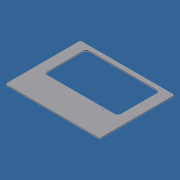
# Autodesk Inventor part: P1699_002_FaceAvant
Saved by Autodesk Inventor 2015 SP2 (Build 190223200, 223)
## iProperties
Created: 2017-01-26
Part Number: P1699_002_FaceAvant
Project: Nom Projet
Material: .
Description: Nom pièce
Document SubType Name: Modeling
Designer: Jean-Marc.VULLIAMY
Authority: brut Ø
Density: 1 g/cm^3
Appearance: Par défaut(1)
Mass: 77.5499 g
Surface Area: 565.1 cm^2
Volume: 77.5499 cm^3
Material number: ---
Author: Jean-Marc.VULLIAMY
Autodesk Inventor part; units mm, degrees
ref_plane "Plan YZ" through (0, 0, 0) normal (1, 0, 0) x (0, 1, 0)
ref_plane "Plan XZ" through (0, 0, 0) normal (0, 1, 0) x (-1, 0, 0)
ref_plane "Plan XY" through (0, 0, 0) normal (0, 0, 1) x (1, 0, 0)
sketch "Esquisse1" plane through (0, 0, 0) normal (0, 0, 1) x (1, 0, 0)
  line L0 (-88.5, 55.5) -> (88.5, 55.5)
  line L1 (96.5, 47.5) -> (96.5, -47.5)
  line L2 (88.5, -55.5) -> (-88.5, -55.5)
  line L3 (-96.5, -47.5) -> (-96.5, 47.5)
  line L4 (-170.8, 0) -> (170.8, 0) construction
  line L5 (0, -167.3) -> (0, 104.3) construction
  arc A0 (-88.5, 55.5) -> (-96.5, 47.5) centre (-88.5, 47.5) ccw
  arc A1 (-96.5, -47.5) -> (-88.5, -55.5) centre (-88.5, -47.5) ccw
  arc A2 (88.5, -55.5) -> (96.5, -47.5) centre (88.5, -47.5) ccw
  arc A3 (96.5, 47.5) -> (88.5, 55.5) centre (88.5, 47.5) ccw
  line L6 (-83.4, 49.1) -> (86.6, 49.1) construction
  line L7 (86.6, 49.1) -> (86.6, -51.9) construction
  line L8 (86.6, -51.9) -> (-83.4, -51.9) construction
  line L9 (-83.4, -51.9) -> (-83.4, 49.1) construction
  line L10 (88.5, 52.5) -> (-88.5, 52.5)
  arc A4 (-88.5, 52.5) -> (-93.5, 47.5) centre (-88.5, 47.5) ccw
  line L11 (-93.5, 47.5) -> (-93.5, -47.5)
  arc A5 (-93.5, -47.5) -> (-88.5, -52.5) centre (-88.5, -47.5) ccw
  line L12 (-88.5, -52.5) -> (88.5, -52.5)
  arc A6 (88.5, -52.5) -> (93.5, -47.5) centre (88.5, -47.5) ccw
  line L13 (93.5, -47.5) -> (93.5, 47.5)
  arc A7 (93.5, 47.5) -> (88.5, 52.5) centre (88.5, 47.5) ccw
  line L14 (-122, 65.5) -> (122, 65.5)
  line L15 (122, 65.5) -> (122, -128.5)
  line L16 (122, -128.5) -> (-122, -128.5)
  line L17 (-122, -128.5) -> (-122, 65.5)
  line L18 (122, -31.5) -> (-122, -31.5) construction
  point P0 (0, 0)
  point P1 (-96.5, 55.5)
  point P2 (96.5, -55.5)
  point P3 (96.5, 55.5)
  point P4 (-62.24, 33.92)
  point P5 (-62.24, -31.73)
  point P6 (63.96, -31.73)
  point P7 (63.96, 33.92)
  point P8 (-62.24, 60.5)
  point P9 (-62.24, -60.5)
  point P10 (63.96, -60.5)
  point P11 (63.96, 60.5)
  point P12 (-117, -123.5)
  point P13 (0, -123.5)
  point P14 (117, -123.5)
  point P15 (-117, -31.5)
  point P16 (0, -31.5)
  point P17 (117, -31.5)
  point P18 (-117, 60.5)
  point P19 (0, 60.5)
  point P20 (117, 60.5)
  dimension "d0" = 193
  dimension "d1" = 111
  dimension "d2" = 8
  dimension "d3" = 170
  dimension "d4" = 101
  dimension "d6" = 6.4
  dimension "d7" = 9.9
  dimension "d8" = 32.54
  dimension "d9" = 21.58
  dimension "d10" = 126.2
  dimension "d11" = 65.65
  dimension "d12" = 121
  dimension "d13" = 3
  dimension "d14" = 244
  dimension "d15" = 194
  dimension "d39" = 10
  dimension "d42" = 117
  dimension "d45" = 92
  constraints: 34 end point, 16 point on circle, 8 centre point, 8 parallel, 8 tangent, 6 point on line, 4 horizontal, 4 horizontal alignment, 4 midpoint, 4 perpendicular, 4 vertical alignment, 3 equal radius, 2 symmetric about line, 1 vertical, 18 other
  measures "d0" distance of point (-96.5, 55.5) point (96.5, 55.5)
  measures "d1" distance of point (96.5, 55.5) point (96.5, -55.5)
  measures "d2" radius of A0
  measures "d3" distance of L6.start L6.end
  measures "d4" distance of L6.end L7.end
  measures "d6" distance between parallel lines of L0 L6
  measures "d7" distance between parallel lines of L1 L7
  measures "d8" distance from line of L1 point (63.96, 33.92)
  measures "d9" distance from line of L0 point (63.96, 33.92)
  measures "d10" distance of point (-62.24, 33.92) point (63.96, 33.92)
  measures "d11" distance of point (63.96, -31.73) point (63.96, 33.92)
  measures "d12" distance of point (-62.24, -60.5) point (-62.24, 60.5)
  measures "d13" distance between parallel lines of L2 L12
  measures "d14" distance of L14.start L14.end
  measures "d15" distance of L14.end L15.end
  measures "d39" distance between parallel lines of L0 L14
  measures "d42" distance of point (-117, -123.5) point (0, -123.5)
  measures "d45" distance of point (-117, -123.5) point (-117, -31.5)
extrude "Extrusion1" add sketch "Esquisse1" along normal blind 3 contours L14 L15 L16 L17
hole "Perçage6" at (-62.24, 33.92, 0) at (-62.24, -31.73, 0) at (63.96, -31.73, 0) at (63.96, 33.92, 0) at (-62.24, 60.5, 0) at (-62.24, -60.5, 0) at (63.96, -60.5, 0) at (63.96, 60.5, 0) at (-117, -123.5, 0) at (0, -123.5, 0) at (117, -123.5, 0) at (-117, -31.5, 0) at (0, -31.5, 0) at (117, -31.5, 0) at (-117, 60.5, 0) at (0, 60.5, 0) at (117, 60.5, 0) direction (0, 0, 1) diameter 3.3 end through all
fillet "Congé1" radius 3 4 edges at (122, -128.5, 1.5) (122, 65.5, 1.5) (-122, 65.5, 1.5) (-122, -128.5, 1.5)
sketch "Esquisse9" plane through (0, 0, 3) normal (0, 0, 1) x (1, 0, 0)
  point P0 (0, 0)
  point P1 (-16, -123)
  point P2 (-16, -64)
  dimension "d66" = 59
  dimension "d67" = 64
  dimension "d68" = 16
  constraints: 1 vertical alignment
  measures "d66" distance of point (-16, -64) point (-16, -123)
  measures "d67" vertical distance of point (0, 0) point (-16, -64)
  measures "d68" horizontal distance of point (0, 0) point (-16, -64)
hole "Perçage4" at (-16, -123, 3) at (-16, -64, 3) direction (0, 0, -1) diameter 2.2 end through all
